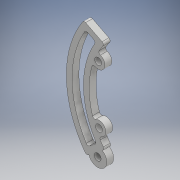
# Autodesk Inventor part: Reverse Gear Link 1 updated
Saved by Autodesk Inventor 2017 (Build 210142000, 142)
## iProperties
Created: 2018-11-20
Part Number: Reverse Gear Link 1 updated
Material: Generic
Document SubType Name: Modeling
Designer: Arman Grewal
Density: 1 g/cm^3
Appearance: Default
Author: Arman Grewal
Autodesk Inventor part; units mm, degrees
ref_plane "YZ Plane" through (0, 0, 0) normal (1, 0, 0) x (0, 1, 0)
ref_plane "XZ Plane" through (0, 0, 0) normal (0, 1, 0) x (-1, 0, 0)
ref_plane "XY Plane" through (0, 0, 0) normal (0, 0, 1) x (1, 0, 0)
sketch "Sketch1" plane through (0, 0, 0) normal (0, 1, 0) x (-1, 0, 0)
  arc A0 (34.7717, -25.2969) -> (36.6925, 22.4201) centre (0, 0) ccw
  circle A1 centre (28.6854, -13.0153) radius 1.5
  circle A2 centre (29.0479, 12.1849) radius 1.5
  line L0 (33.6483, 20.8328) -> (30.9628, 19.4812)
  arc A3 (32.7365, 13.7321) -> (30.5518, 18.0787) centre (0, 0) ccw
  arc A4 (37.3473, 15.6662) -> (34.9611, 20.4443) centre (0, 0) ccw
  arc A5 (34.9611, 20.4443) -> (33.6483, 20.8328) centre (34.0979, 19.9395) ccw
  arc A6 (30.9628, 19.4812) -> (30.5518, 18.0787) centre (31.4124, 18.5879) ccw
  line L1 (34.5435, 24.12) -> (27.3337, 20.4914)
  arc A7 (34.3646, 21.4319) -> (33.0708, 23.3788) centre (0, 0) ccw
  arc A8 (27.7564, 17.8489) -> (26.9661, 19.0218) centre (0, 0) ccw
  arc A9 (27.3337, 20.4914) -> (26.9661, 19.0218) centre (27.7833, 19.5982) ccw
  arc A10 (36.6925, 22.4201) -> (35.8263, 23.7798) centre (0, 0) ccw
  arc A11 (35.8263, 23.7798) -> (34.5435, 24.12) centre (34.9931, 23.2268) ccw
  circle A12 centre (29.253, -24.2541) radius 1.5
  arc A13 (27.2186, -20.8101) -> (33.1098, -25.315) centre (29.253, -24.2541) ccw
  arc A14 (28.0626, 15.0184) -> (30.379, 9.4963) centre (29.0479, 12.1849) ccw
  arc A15 (28.6009, 16.4618) -> (27.7564, 17.8489) centre (0, 0) ccw
  arc A16 (30.0933, -10.3662) -> (27.619, -15.8194) centre (28.6854, -13.0153) ccw
  arc A17 (31.5176, -9.7795) -> (31.7859, 8.8689) centre (0, 0) ccw
  arc A18 (26.7939, -19.2636) -> (28.1155, -17.2777) centre (0, 0) ccw
  arc A19 (30.0933, -10.3662) -> (31.5176, -9.7795) centre (30.5625, -9.4832) ccw
  arc A20 (28.1155, -17.2777) -> (27.619, -15.8194) centre (27.2635, -16.7541) ccw
  arc A21 (31.7859, 8.8689) -> (30.379, 9.4963) centre (30.8227, 8.6001) ccw
  arc A22 (28.0626, 15.0184) -> (28.6009, 16.4618) centre (27.7342, 15.963) ccw
  arc A23 (33.3556, -25.5029) -> (34.7717, -25.2969) centre (33.963, -24.7086) ccw
  arc A24 (26.7939, -19.2636) -> (26.9984, -20.6418) centre (27.6058, -19.8474) ccw
  arc A25 (34.2723, -21.5792) -> (33.0708, 23.3788) centre (0, 0) ccw
  arc A26 (30.182, -18.6894) -> (30.5518, 18.0787) centre (0, 0) ccw
  line L2 (32.8186, -21.8408) -> (30.4248, -20.0103)
  arc A27 (32.8186, -21.8408) -> (34.2723, -21.5792) centre (33.426, -21.0464) ccw
  arc A28 (30.182, -18.6894) -> (30.4248, -20.0103) centre (31.0322, -19.2159) ccw
  line L3 (33.3556, -25.5029) -> (33.1098, -25.315)
  line L4 (30.1876, -23.0805) -> (30.1642, -23.0625)
  line L5 (27.2186, -20.8101) -> (26.9984, -20.6418)
  point P0 (26.2158, -20.0433)
  point P1 (29.6958, -19.4528)
  dimension "d2" = 3
  dimension "d0" = 1
  dimension "d1" = 8
  dimension "d3" = 3
  dimension "d4" = 43
  dimension "d5" = 33
  dimension "d6" = 33
  dimension "d7" = 2.5339
  dimension "d8" = 3.4819
  dimension "d9" = 29.0479
  dimension "d10" = 1
  dimension "d11" = 1
  dimension "d12" = 40.5
  dimension "d13" = 1
  dimension "d14" = 1
  dimension "d15" = 43
  dimension "d16" = 40.5
  dimension "d17" = 35.5
  dimension "d18" = 64.12
  dimension "d19" = 2.5829
  dimension "d20" = 0.0025
  dimension "d21" = 35.1283
  dimension "d22" = 6.2779
  dimension "d23" = 40.0956
  dimension "d24" = 0.0494
  dimension "d25" = 37.8965
  dimension "d26" = 40.9793
  dimension "d27" = 30.7911
  dimension "d28" = 9.8494
  dimension "d29" = 8.7909
  dimension "d30" = 37.6697
  dimension "d31" = 0.0165
  dimension "d32" = 0
  dimension "d33" = 6.0158
  dimension "d34" = 0.0025
  constraints: 56 point on circle, 37 tangent, 28 centre point, 12 end point, 9 equal radius, 5 coincident, 4 concentric, 2 parallel, 2 point on line, 7 other
  measures "d0" radius of A11
  measures "d1" diameter of A13
  measures "d3" radius of A14
  measures "d4" radius of A0
  measures "d5" radius of A18
  measures "d6" radius of A17
  measures "d7" distance between parallel lines of L0 L1
  measures "d8" distance from line of point (0, 0) L0
  measures "d9" horizontal distance of A15.centre A14.centre
  measures "d10" radius of A19
  measures "d11" radius of A23
  measures "d12" radius of A4
  measures "d13" radius of A27
  measures "d14" radius of A28
  measures "d15" radius of A10
  measures "d16" radius of A7
  measures "d17" radius of A3
  measures "d18" angle of L3 L0
  measures "d19" distance between parallel lines of L3 L2
  measures "d20" distance from line of point (0, 0) L5
  measures "d21" distance from line of A4.start L5
  measures "d22" distance from line of A4.start L0
  measures "d23" distance from line of A0.end L5
  measures "d24" distance from line of A0.end L0
  measures "d25" distance from line of A7.start L5
  measures "d26" distance from line of L3.end L0
  measures "d27" distance from line of A3.start L5
  measures "d28" distance from line of A21.start L0
  measures "d29" distance from line of A19.end L2
  measures "d30" distance from line of L4.start L0
  measures "d31" distance from line of A15.end L0
  measures "d32" distance from line of point (26.216, -20.043) L5
  measures "d33" distance from line of point (0, 0) L1
  measures "d34" distance from line of point (0, 0) L4
extrude "Extrusion1" add sketch "Sketch1" along normal blind 3
body "Solid1"
